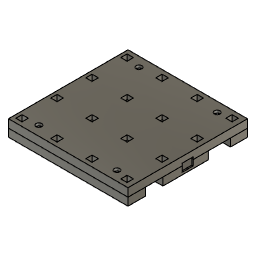
housing-ledrunner (Autodesk Fusion 360 design; units mm, degrees)
Autodesk Fusion 360 part; units mm, degrees
note: some values were not read from the file. Set by a fixed rule: which face or edge a step refers to.
sketch "Sketch1" plane through (0, 0, 0) normal (0, 0, 1) x (1, 0, 0)
  line L0 (-63.5, 63.5) -> (63.5, 63.5)
  line L1 (63.5, 63.5) -> (63.5, -63.5)
  line L2 (63.5, -63.5) -> (-63.5, -63.5)
  line L3 (-63.5, -63.5) -> (-63.5, 63.5)
  line L4 (-63.5, 63.5) -> (63.5, -63.5) construction
  line L5 (-42.5, 54.5) -> (42.5, 54.5) construction
  line L6 (-42.5, 54.5) -> (-42.5, -54.5) construction
  circle A0 centre (-42.5, 54.5) radius 1.8
  circle A1 centre (42.5, 54.5) radius 1.8
  circle A2 centre (42.5, -54.5) radius 1.8
  circle A3 centre (-42.5, -54.5) radius 1.8
  circle A4 centre (-42.5, 54.5) radius 3.1
  circle A5 centre (42.5, 54.5) radius 3.1
  circle A6 centre (42.5, -54.5) radius 3.1
  circle A7 centre (-42.5, -54.5) radius 3.1
  line L7 (-62.5, 61.5) -> (62.5, 61.5) construction
  line L8 (62.5, 61.5) -> (62.5, -61.5) construction
  line L9 (62.5, -61.5) -> (-62.5, -61.5) construction
  line L10 (-62.5, -61.5) -> (-62.5, 61.5) construction
  line L11 (-62.5, 61.5) -> (62.5, -61.5) construction
  line L12 (65, -65) -> (-65, -65)
  line L13 (-65, -65) -> (-65, 65)
  line L14 (-65, 65) -> (65, 65)
  line L15 (65, 65) -> (65, -65)
  line L16 (49.5, -49.5) -> (-49.5, -49.5)
  line L17 (-49.5, -49.5) -> (-49.5, 49.5)
  line L18 (-49.5, 49.5) -> (49.5, 49.5)
  line L19 (49.5, 49.5) -> (49.5, -49.5)
  line L20 (-61.55, 60.55) -> (-54.75, 60.55)
  line L21 (-54.75, 60.55) -> (-54.75, 53.75)
  line L22 (-54.75, 53.75) -> (-61.55, 53.75)
  line L23 (-61.55, 53.75) -> (-61.55, 60.55)
  line L24 (-16.65, 53.75) -> (-23.45, 53.75)
  line L25 (-16.65, 60.55) -> (-16.65, 53.75)
  line L26 (-23.45, 53.75) -> (-23.45, 60.55)
  line L27 (-23.45, 60.55) -> (-16.65, 60.55)
  line L28 (21.45, 53.75) -> (14.65, 53.75)
  line L29 (21.45, 60.55) -> (21.45, 53.75)
  line L30 (14.65, 53.75) -> (14.65, 60.55)
  line L31 (14.65, 60.55) -> (21.45, 60.55)
  line L32 (59.55, 53.75) -> (52.75, 53.75)
  line L33 (59.55, 60.55) -> (59.55, 53.75)
  line L34 (52.75, 53.75) -> (52.75, 60.55)
  line L35 (52.75, 60.55) -> (59.55, 60.55)
  line L36 (21.45, 22.45) -> (21.45, 15.65)
  line L37 (59.55, 22.45) -> (59.55, 15.65)
  line L38 (-61.55, 22.45) -> (-54.75, 22.45)
  line L39 (-54.75, 15.65) -> (-61.55, 15.65)
  line L40 (52.75, 22.45) -> (59.55, 22.45)
  line L41 (21.45, 15.65) -> (14.65, 15.65)
  line L42 (52.75, 15.65) -> (52.75, 22.45)
  line L43 (-23.45, 22.45) -> (-16.65, 22.45)
  line L44 (-54.75, 22.45) -> (-54.75, 15.65)
  line L45 (14.65, 22.45) -> (21.45, 22.45)
  line L46 (14.65, 15.65) -> (14.65, 22.45)
  line L47 (59.55, 15.65) -> (52.75, 15.65)
  line L48 (-61.55, 15.65) -> (-61.55, 22.45)
  line L49 (-16.65, 15.65) -> (-23.45, 15.65)
  line L50 (-16.65, 22.45) -> (-16.65, 15.65)
  line L51 (-23.45, 15.65) -> (-23.45, 22.45)
  line L52 (21.45, -15.65) -> (21.45, -22.45)
  line L53 (59.55, -15.65) -> (59.55, -22.45)
  line L54 (-61.55, -15.65) -> (-54.75, -15.65)
  line L55 (-54.75, -22.45) -> (-61.55, -22.45)
  line L56 (52.75, -15.65) -> (59.55, -15.65)
  line L57 (21.45, -22.45) -> (14.65, -22.45)
  line L58 (52.75, -22.45) -> (52.75, -15.65)
  line L59 (-23.45, -15.65) -> (-16.65, -15.65)
  line L60 (-54.75, -15.65) -> (-54.75, -22.45)
  line L61 (14.65, -15.65) -> (21.45, -15.65)
  line L62 (14.65, -22.45) -> (14.65, -15.65)
  line L63 (59.55, -22.45) -> (52.75, -22.45)
  line L64 (-61.55, -22.45) -> (-61.55, -15.65)
  line L65 (-16.65, -22.45) -> (-23.45, -22.45)
  line L66 (-16.65, -15.65) -> (-16.65, -22.45)
  line L67 (-23.45, -22.45) -> (-23.45, -15.65)
  line L68 (21.45, -53.75) -> (21.45, -60.55)
  line L69 (59.55, -53.75) -> (59.55, -60.55)
  line L70 (-61.55, -53.75) -> (-54.75, -53.75)
  line L71 (-54.75, -60.55) -> (-61.55, -60.55)
  line L72 (52.75, -53.75) -> (59.55, -53.75)
  line L73 (21.45, -60.55) -> (14.65, -60.55)
  line L74 (52.75, -60.55) -> (52.75, -53.75)
  line L75 (-23.45, -53.75) -> (-16.65, -53.75)
  line L76 (-54.75, -53.75) -> (-54.75, -60.55)
  line L77 (14.65, -53.75) -> (21.45, -53.75)
  line L78 (14.65, -60.55) -> (14.65, -53.75)
  line L79 (59.55, -60.55) -> (52.75, -60.55)
  line L80 (-61.55, -60.55) -> (-61.55, -53.75)
  line L81 (-16.65, -60.55) -> (-23.45, -60.55)
  line L82 (-16.65, -53.75) -> (-16.65, -60.55)
  line L83 (-23.45, -60.55) -> (-23.45, -53.75)
  line L84 (-16.65, 15.65) -> (14.65, -15.65) construction
  line L85 (49.5, -6) -> (65, -6)
  line L86 (65, -6) -> (65, 6)
  line L87 (65, 6) -> (49.5, 6)
  line L88 (49.5, 6) -> (49.5, -6)
  line L89 (42.5, 54.5) -> (42.5, -54.5) construction
  line L90 (-42.5, -54.5) -> (42.5, -54.5) construction
  line L91 (-42.5, -54.5) -> (42.5, 54.5) construction
  line L92 (-58.15, 15.65) -> (-58.15, -15.65) construction
  line L93 (-58.15, 0) -> (-1, 0) construction
  point P0 (-42.5, 54.5)
  point P1 (42.5, 54.5)
  point P2 (42.5, -54.5)
  point P3 (-42.5, -54.5)
  point P4 (-1, 0)
  point P5 (65, 0)
  point P6 (65, 0)
  point P7 (-58.15, 0)
  dimension "d1" = 127
  dimension "d2" = 127
  dimension "d3" = 85
  dimension "d4" = 109
  dimension "d5" = 3.6
  dimension "d6" = 3.6
  dimension "d7" = 3.6
  dimension "d8" = 3.6
  dimension "d9" = 6.2
  dimension "d13" = 125
  dimension "d14" = 123
  dimension "d15" = -1.5
  dimension "d21" = 14
  dimension "d25" = 6.8
  dimension "d26" = 6.8
  dimension "d29" = 114.3
  dimension "d30" = 0
  dimension "d33" = 0
  dimension "d34" = -114.3
  dimension "d37" = 12
  dimension "d42" = 130
  dimension "d43" = 130
  dimension "d45" = 20
  dimension "d46" = 7
  dimension "d84" = 1
  constraint horizontal L0
  constraint vertical L1
  constraint horizontal L2
  constraint vertical L3
  constraint coincident P1 L5.end
  constraint coincident P0 L5.start
  constraint parallel L0 L5
  constraint coincident P3 L6.end
  constraint parallel L3 L6
  constraint coincident P2 A2.centre
  constraint concentric A0 A4
  constraint horizontal L7
  constraint vertical L8
  constraint horizontal L9
  constraint vertical L10
  constraint horizontal L20
  constraint vertical L21
  constraint horizontal L22
  constraint vertical L23
  constraint midpoint L84 P4
  constraint horizontal L85
  constraint vertical L86
  constraint horizontal L87
  constraint vertical L88
  constraint midpoint L15 P6
  constraint midpoint L86 P6
  constraint coincident P6 P5
  constraint coincident L19 L85.start
  constraint midpoint L4 origin
  constraint midpoint L11 origin
  constraint parallel L5 L90
  constraint parallel L6 L89
  constraint equal A4 A7
  constraint equal A4 A5
  constraint equal A5 A6
  constraint midpoint L39 L92.start
  constraint midpoint L54 L92.end
  constraint midpoint L92 P7
  constraint coincident P7 L93.start
  constraint coincident P4 L93.end
  constraint coincident origin L93
  measures "d1" distance of L0.start L0.end
  measures "d2" distance of L0.start L2.end
  measures "d3" distance of P0 P1
  measures "d4" distance of P0 P3
  measures "d5" diameter of A0
  measures "d6" diameter of A1
  measures "d7" diameter of A2
  measures "d8" diameter of A3
  measures "d9" diameter of A4
  measures "d13" distance of L7.start L7.end
  measures "d14" distance of L7.start L9.end
  measures "d25" distance of L20.start L20.end
  measures "d26" distance of L20.start L22.end
  measures "d37" distance of L85 L87
  measures "d42" distance of L13.end L14.end
  measures "d43" distance of L12.start L14.end
  measures "d45" distance of P1 L8
  measures "d46" distance of P1 L7
  measures "d84" horizontal distance of P4 origin
extrude "Extrude1" add sketch "Sketch1" along normal blind 7.3 contours L0 L1 L2 L3 L12 L13 L14 L15 L85 L87 | L0 L1 L2 L3 L16 L17 L18 L19 L85 L87 | L1 L15 L85 L86 L87 | L1 L19 L85 L87 L88 | L16 L17 L18 L19 L88 | A4 | A5 | A6 | A7 | L20 L21 L22 L23 | L24 L25 L26 L27 | L28 L29 L30 L31 | L32 L33 L34 L35 | L36 L41 L45 L46 | L37 L40 L42 L47 | L38 L39 L44 L48 | L43 L49 L50 L51 | L52 L57 L61 L62 | L53 L56 L58 L63 | L54 L55 L60 L64 | L59 L65 L66 L67 | L68 L73 L77 L78 | L69 L72 L74 L79 | L70 L71 L76 L80 | L75 L81 L82 L83 makes body 1
extrude "Extrude2" cut sketch "Sketch1" against normal blind 2.8 from surface at 7.3 contours A4 | A5 | A6 | A7 bodies 1
extrude "Extrude3" cut sketch "Sketch1" along normal blind 2.5 contours L16 L17 L18 L19 L88 | L36 L41 L45 L46 | L43 L49 L50 L51 | L52 L57 L61 L62 | L59 L65 L66 L67 bodies 1
chamfer "Chamfer1" distance 2.5 angle 45 4 edges at (0, -49.5, 0) (-49.5, 0, 0) (49.5, 0, 0) (0, 49.5, 0) on bodies 1
extrude "Extrude4" cut sketch "Sketch1" along normal up to surface (7.3 mm away) contours L20 L21 L22 L23 | L24 L25 L26 L27 | L28 L29 L30 L31 | L32 L33 L34 L35 | L36 L41 L45 L46 | L37 L40 L42 L47 | L38 L39 L44 L48 | L43 L49 L50 L51 | L52 L57 L61 L62 | L53 L56 L58 L63 | L54 L55 L60 L64 | L59 L65 L66 L67 | L68 L73 L77 L78 | L69 L72 L74 L79 | L70 L71 L76 L80 | L75 L81 L82 L83 bodies 1
extrude "Extrude5" add sketch "Sketch1" against normal blind 1.6 contours L0 L1 L2 L3 L12 L13 L14 L15 L85 L87 bodies 1
extrude "Extrude6" cut sketch "Sketch1" along normal blind 1 contours L1 L15 L85 L86 L87 | L1 L19 L85 L87 L88 bodies 1
chamfer "Chamfer2" distance 1 angle 45 4 edges at (40.8218, 53.8491, 4.5) (-44.1782, 53.8491, 4.5) (40.8218, -55.1509, 4.5) (-44.1782, -55.1509, 4.5) on bodies 1
sketch "Sketch2" plane through (0, 0, -1.6) normal (0, 0, -1) x (1, 0, 0)
  line L0 (63.5, 63.5) -> (63.5, 6)
  line L1 (63.5, 6) -> (65, 6)
  line L2 (65, 6) -> (65, 65)
  line L3 (65, 65) -> (-65, 65)
  line L4 (-65, 65) -> (-65, -65)
  line L5 (-65, -65) -> (65, -65)
  line L6 (65, -65) -> (65, -6)
  line L7 (65, -6) -> (63.5, -6)
  line L8 (63.5, -6) -> (63.5, -63.5)
  line L9 (63.5, -63.5) -> (-63.5, -63.5)
  line L10 (-63.5, -63.5) -> (-63.5, 63.5)
  line L11 (-63.5, 63.5) -> (63.5, 63.5)
  line L12 (62.5, 43) -> (47.5, 43)
  line L13 (47.5, 43) -> (47.5, 30)
  line L14 (47.5, 30) -> (62.5, 30)
  line L15 (62.5, 30) -> (62.5, 43)
  line L16 (62.5, -25.5) -> (47.5, -25.5)
  line L17 (47.5, -25.5) -> (47.5, -43.5)
  line L18 (47.5, -43.5) -> (62.5, -43.5)
  line L19 (62.5, -43.5) -> (62.5, -25.5)
  line L20 (62.5, -61.5) -> (62.5, 61.5)
  line L21 (62.5, 61.5) -> (-62.5, 61.5)
  line L22 (-65, 65) -> (65, 65)
  line L23 (65, 65) -> (65, -65)
  line L24 (65, -65) -> (-65, -65)
  line L25 (-65, -65) -> (-65, 65)
  line L26 (-63.5, 63.5) -> (63.5, 63.5)
  line L27 (63.5, 63.5) -> (63.5, -63.5)
  line L28 (63.5, -63.5) -> (-63.5, -63.5)
  line L29 (-63.5, -63.5) -> (-63.5, 63.5)
  line L30 (62.5, -25.5) -> (63.5, -25.5)
  line L31 (63.5, -25.5) -> (63.5, -43.5)
  line L32 (63.5, -43.5) -> (62.5, -43.5)
  line L33 (62.5, -43.5) -> (62.5, -25.5)
  line L34 (62.5, 43) -> (63.5, 43)
  line L35 (63.5, 43) -> (63.5, 30)
  line L36 (63.5, 30) -> (62.5, 30)
  line L37 (62.5, 30) -> (62.5, 43)
  arc A0 (50.5, 46) -> (47.5, 43) centre (50.5, 43) ccw
  line L38 (50.5, 43) -> (50.5, 46) construction
  line L39 (50.5, 43) -> (47.5, 43) construction
  arc A1 (47.5, 30) -> (50.5, 27) centre (50.5, 30) ccw
  line L40 (50.5, 30) -> (47.5, 30) construction
  line L41 (50.5, 30) -> (50.5, 27) construction
  arc A2 (50.5, -22.5) -> (47.5, -25.5) centre (50.5, -25.5) ccw
  line L42 (50.5, -25.5) -> (50.5, -22.5) construction
  line L43 (50.5, -25.5) -> (47.5, -25.5) construction
  arc A3 (47.5, -43.5) -> (50.5, -46.5) centre (50.5, -43.5) ccw
  line L44 (50.5, -43.5) -> (47.5, -43.5) construction
  line L45 (50.5, -43.5) -> (50.5, -46.5) construction
  line L46 (50.5, -22.5) -> (65, -22.5)
  line L47 (50.5, -46.5) -> (65, -46.5)
  line L48 (50.5, 46) -> (65, 46)
  line L49 (50.5, 27) -> (65, 27)
  line L50 (49.5, -6) -> (65, -6)
  line L51 (65, -6) -> (65, 6)
  line L52 (65, 6) -> (49.5, 6)
  line L53 (49.5, 6) -> (49.5, -6)
  line L54 (50.5, 25.5) -> (65, 25.5)
  arc A4 (46, 30) -> (50.5, 25.5) centre (50.5, 30) ccw
  line L55 (46, 43) -> (46, 30)
  arc A5 (50.5, 47.5) -> (46, 43) centre (50.5, 43) ccw
  line L56 (50.5, 47.5) -> (65, 47.5)
  line L57 (50.5, -21) -> (65, -21)
  arc A6 (50.5, -21) -> (46, -25.5) centre (50.5, -25.5) ccw
  line L58 (46, -25.5) -> (46, -43.5)
  arc A7 (46, -43.5) -> (50.5, -48) centre (50.5, -43.5) ccw
  line L59 (50.5, -48) -> (65, -48)
  line L60 (-47, -59) -> (-38, -59)
  line L61 (-38, -59) -> (-38, -50)
  line L62 (-38, -50) -> (-47, -50)
  line L63 (-47, -50) -> (-47, -59)
  line L64 (38, -50) -> (47, -50)
  line L65 (47, -50) -> (47, -59)
  line L66 (47, -59) -> (38, -59)
  line L67 (38, -59) -> (38, -50)
  line L68 (38, 50) -> (47, 50)
  line L69 (47, 50) -> (47, 59)
  line L70 (47, 59) -> (38, 59)
  line L71 (38, 59) -> (38, 50)
  line L72 (-47, 50) -> (-38, 50)
  line L73 (-38, 50) -> (-38, 59)
  line L74 (-38, 59) -> (-47, 59)
  line L75 (-47, 59) -> (-47, 50)
  line L76 (-47, -50) -> (-38, -59) construction
  line L77 (38, 59) -> (47, 50) construction
  line L78 (-45.5, 57.5) -> (-45.5, 51.5)
  line L79 (-45.5, 51.5) -> (-39.5, 51.5)
  line L80 (-39.5, 51.5) -> (-39.5, 57.5)
  line L81 (-39.5, 57.5) -> (-45.5, 57.5)
  line L82 (39.5, 51.5) -> (45.5, 51.5)
  line L83 (45.5, 51.5) -> (45.5, 57.5)
  line L84 (45.5, 57.5) -> (39.5, 57.5)
  line L85 (39.5, 57.5) -> (39.5, 51.5)
  line L86 (45.5, -57.5) -> (39.5, -57.5)
  line L87 (39.5, -57.5) -> (39.5, -51.5)
  line L88 (39.5, -51.5) -> (45.5, -51.5)
  line L89 (45.5, -51.5) -> (45.5, -57.5)
  line L90 (-45.5, -51.5) -> (-45.5, -57.5)
  line L91 (-45.5, -57.5) -> (-39.5, -57.5)
  line L92 (-39.5, -57.5) -> (-39.5, -51.5)
  line L93 (-39.5, -51.5) -> (-45.5, -51.5)
  circle A8 centre (42.5, -54.5) radius 1.8
  circle A9 centre (-42.5, -54.5) radius 1.8
  circle A10 centre (-42.5, 54.5) radius 1.8
  circle A11 centre (42.5, 54.5) radius 1.8
  circle A12 centre (42.5, 54.5) radius 1.8
  circle A13 centre (-42.5, 54.5) radius 1.8
  circle A14 centre (-42.5, -54.5) radius 1.8
  circle A15 centre (42.5, -54.5) radius 1.8
  line L94 (47.5, 30) -> (46, 30)
  line L95 (47.5, 43) -> (46, 43)
  line L96 (47.5, -43.5) -> (46, -43.5)
  line L97 (47.5, -25.5) -> (46, -25.5)
  point P0 (62.5, 36.5)
  point P1 (62.5, -34.5)
  point P2 (49.5, -6)
  point P3 (49.5, -6)
  point P4 (-42.5, -54.5)
  point P5 (42.5, -54.5)
  point P6 (42.5, 54.5)
  point P7 (-42.5, 54.5)
  point P8 (-42.5, 54.5)
  point P9 (42.5, 54.5)
  point P10 (42.5, -54.5)
  point P11 (-42.5, -54.5)
  point P12 (-42.5, -54.5)
  point P13 (42.5, 54.5)
  dimension "d47" = 13
  dimension "d48" = 18
  dimension "d49" = 15
  dimension "d53" = 27
  dimension "d54" = 25
  dimension "d55" = 90
  dimension "d56" = 90
  dimension "d57" = 90
  dimension "d58" = 90
  dimension "d59" = 3
  dimension "d62" = 1.5
  dimension "d63" = 1.5
  dimension "d67" = 9
  dimension "d68" = 9
  dimension "d69" = -1.5
  dimension "d70" = 6
  dimension "d71" = -1.5
  dimension "d72" = 1.5
  dimension "d73" = -1.5
  constraint horizontal L12
  constraint vertical L13
  constraint horizontal L14
  constraint vertical L15
  constraint horizontal L16
  constraint vertical L17
  constraint horizontal L18
  constraint vertical L19
  constraint coincident L16.start L20
  constraint coincident L12.start L20
  constraint horizontal L22
  constraint vertical L23
  constraint horizontal L24
  constraint vertical L25
  constraint coincident L5.end L6.start
  constraint coincident L3.end L4.start
  constraint horizontal L26
  constraint vertical L27
  constraint horizontal L28
  constraint vertical L29
  constraint coincident L8.end L9.start
  constraint coincident L10.end L11.start
  constraint horizontal L30
  constraint vertical L31
  constraint horizontal L32
  constraint vertical L33
  constraint horizontal L34
  constraint vertical L35
  constraint horizontal L36
  constraint vertical L37
  constraint collinear L14 L36
  constraint collinear L18 L32
  constraint coincident L27 L30.end
  constraint coincident L27 L34.end
  constraint midpoint L37 P0
  constraint midpoint L33 P1
  constraint coincident L12 A0.centre
  constraint coincident L14 A1.centre
  constraint coincident L16 A2.centre
  constraint coincident L18 A3.centre
  constraint coincident L23 L46.end
  constraint coincident L23 L47.end
  constraint coincident L23 L48.end
  constraint coincident L23 L49.end
  constraint parallel L12 L48
  constraint parallel L14 L49
  constraint parallel L16 L46
  constraint parallel L18 L47
  constraint equal A2 A3
  constraint equal A1 A2
  constraint equal A0 A1
  constraint coincident P3 P2
  constraint horizontal L50
  constraint vertical L51
  constraint horizontal L52
  constraint vertical L53
  constraint coincident L1.end L2.start
  constraint equal L12 L16
  constraint coincident P8 P7
  constraint coincident P13 P9
  constraint coincident P10 P5
  constraint coincident P12 P11
  constraint horizontal L60
  constraint vertical L61
  constraint horizontal L62
  constraint vertical L63
  constraint horizontal L64
  constraint vertical L65
  constraint horizontal L66
  constraint vertical L67
  constraint horizontal L68
  constraint vertical L69
  constraint horizontal L70
  constraint vertical L71
  constraint horizontal L72
  constraint vertical L73
  constraint horizontal L74
  constraint vertical L75
  constraint midpoint L76 P12
  constraint equal L61 L65
  constraint equal L62 L64
  constraint equal L64 L68
  constraint equal L65 L69
  constraint equal L71 L73
  constraint equal L70 L74
  constraint collinear L62 L64
  constraint collinear L61 L73
  constraint collinear L70 L74
  constraint collinear L67 L71
  constraint midpoint L77 P13
  constraint tangent A11 A12
  constraint equal A10 A13
  constraint equal A9 A14
  constraint equal A8 A15
  measures "d47" distance of L12.start L14.end
  measures "d48" distance of L16.start L18.end
  measures "d49" distance of L12.start L12.end
  measures "d53" distance of L20.start P1
  measures "d54" distance of L20.end P0
  measures "d55" angle of L38 L39
  measures "d56" angle of L40 L41
  measures "d57" angle of L42 L43
  measures "d58" angle of L44 L45
  measures "d59" vertical distance of L18.end L47.end
  measures "d67" distance of L61.end L62.end
  measures "d68" distance of L60.start L62.end
  measures "d70" distance of L78.start L80.end
extrude "Extrude7" add sketch "Sketch2" along normal blind 7 separate body contours L0 L20 L27 L48 L56 | L0 L2 L23 L27 L48 L56 | L0 L2 L23 L27 L49 L54 | L0 L20 L27 L49 L54 | L0 L2 L3 L4 L5 L6 L8 L9 L10 L11 L22 L23 L24 L25 L26 L27 L28 L29 L56 L59 | L20 A0 L48 A5 L56 L95 | L13 L55 L94 L95 | L0 L1 L2 L23 L27 L52 L54 | L20 A1 L49 L54 A4 L94 | L6 L7 L8 L23 L27 L50 L57 | L6 L8 L23 L27 L46 L57 | L8 L20 L27 L46 L57 | L20 A2 L46 L57 A6 L97 | L8 L20 L27 L47 L59 | L6 L8 L23 L27 L47 L59 | L20 A3 L47 A7 L59 L96 | L17 L58 L96 L97 makes body 2
sketch "Sketch3" plane through (65, 0, 0) normal (1, 0, 0) x (0, 1, 0)
  line L0 (-6, -1.6) -> (-27, -1.6)
  line L1 (-27, -1.6) -> (-27, -8.6)
  line L2 (-27, -8.6) -> (-6, -8.6)
  line L3 (-6, -8.6) -> (-6, -1.6)
  line L4 (6, -1.6) -> (-6, -1.6)
  line L5 (-6, -1.6) -> (-6, -7.6)
  line L6 (-6, -7.6) -> (6, -7.6)
  line L7 (6, -7.6) -> (6, -1.6)
  line L8 (6, -7.6) -> (-6, -7.6)
  line L9 (-6, -7.6) -> (-6, -8.6)
  line L10 (-6, -8.6) -> (6, -8.6)
  line L11 (6, -8.6) -> (6, -7.6)
  point P0 (-6, -8.6)
  point P1 (6, -1.6)
  point P2 (6, -1.6)
  dimension "d64" = 6
  constraint coincident P0 L2.end
  constraint coincident P2 P1
  constraint horizontal L4
  constraint vertical L5
  constraint horizontal L6
  constraint vertical L7
  constraint coincident L3 L5.end
  constraint horizontal L8
  constraint vertical L9
  constraint horizontal L10
  constraint vertical L11
  measures "d64" distance of L0.start L5.end
extrude "Extrude8" add sketch "Sketch3" against normal up to surface (1.5 mm away) contours L3 L6 L8 L9 L10 L11 bodies 2
extrude "Extrude9" add sketch "Sketch2" along normal blind 1.5 from surface at 7 contours L0 L20 L27 L48 L56 | L0 L2 L23 L27 L48 L56 | L0 L2 L23 L27 L49 L54 | L0 L20 L27 L49 L54 | L0 L8 L9 L10 L11 L20 L26 L27 L28 L29 L50 L52 L53 L54 A4 L55 A5 L56 L57 A6 L58 A7 L59 | L0 L2 L3 L4 L5 L6 L8 L9 L10 L11 L22 L23 L24 L25 L26 L27 L28 L29 L56 L59 | L20 A0 L48 A5 L56 L95 | L13 L55 L94 L95 | L0 L1 L2 L23 L27 L52 L54 | L0 L20 L27 L52 L54 | L20 A1 L49 L54 A4 L94 | L1 L7 L23 L27 L50 L51 L52 | L20 L27 L50 L52 | L6 L7 L8 L23 L27 L50 L57 | L8 L20 L27 L50 L57 | L20 L50 L52 L53 | L6 L8 L23 L27 L46 L57 | L8 L20 L27 L46 L57 | L20 A2 L46 L57 A6 L97 | L8 L20 L27 L47 L59 | L6 L8 L23 L27 L47 L59 | L20 A3 L47 A7 L59 L96 | L17 L58 L96 L97 | L60 L61 L62 L63 | L64 L65 L66 L67 | L68 L69 L70 L71 | L72 L73 L74 L75 | L78 L79 L80 L81 | L82 L83 L84 L85 | L86 L87 L88 L89 | L90 L91 L92 L93 | A8 A15 | A9 A14 | A10 A13 | A11 A12 bodies 2
extrude "Extrude10" cut sketch "Sketch2" along normal up to surface (8.5 mm away) contours L78 L79 L80 L81 | L82 L83 L84 L85 | L86 L87 L88 L89 | L90 L91 L92 L93 | A8 A15 | A9 A14 | A10 A13 | A11 A12 bodies 2
extrude "Extrude11" add sketch "Sketch2" along normal up to surface (7 mm away) contours L60 L61 L62 L63 | L64 L65 L66 L67 | L68 L69 L70 L71 | L72 L73 L74 L75 bodies 2
extrude "Extrude12" add sketch "Sketch2" along normal blind 4 contours L78 L79 L80 L81 | L82 L83 L84 L85 | L86 L87 L88 L89 | L90 L91 L92 L93 bodies 2
chamfer "Chamfer3" distance 2.4 angle 45 4 edges at (-44.1782, 53.8491, -5.6) (40.8218, 53.8491, -5.6) (40.8218, -55.1509, -5.6) (-44.1782, -55.1509, -5.6) on bodies 2
extrude "Extrude13" cut sketch "Sketch2" along normal blind 3.5 contours L13 L55 L94 L95 | L17 L58 L96 L97 bodies 2
